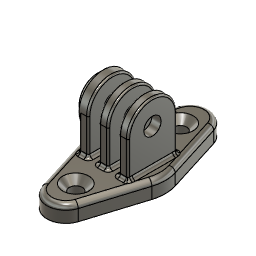
wall_mount (Autodesk Fusion 360 design; units mm, degrees)
Autodesk Fusion 360 part; units mm, degrees
sketch "Sketch3" plane through (0, 0, 0) normal (0, 1, 0) x (1, 0, 0)
  circle A0 centre (0, -16) radius 2
  circle A1 centre (0, 16) radius 2
  line L0 (-7, -16) -> (-12, 0)
  line L1 (-7, 16) -> (-12, 0)
  line L2 (7, -16) -> (12, 0)
  line L3 (7, 16) -> (12, 0)
  line L4 (-7, -16) -> (-5.5086, -20.7724)
  line L5 (7, -16) -> (5.5086, -20.7724)
  line L6 (-7, 16) -> (-5.5086, 20.7724)
  line L7 (7, 16) -> (5.5086, 20.7724)
  arc A2 (5.5086, 20.7724) -> (-5.5086, 20.7724) centre (0, 19.051) ccw
  arc A3 (-5.5086, -20.7724) -> (5.5086, -20.7724) centre (0, -19.051) ccw
  point P0 (0, -18)
  point P1 (0, -14)
  point P2 (0, 14)
  point P3 (0, 18)
  dimension "d1" = 5
  dimension "d2" = 5
  dimension "d3" = 5
  dimension "d4" = 5
  constraint coincident P1 A0
  constraint coincident P0 A0
  constraint coincident P3 A1
  constraint coincident P2 A1
  constraint parallel L0 L4
  constraint parallel L2 L5
  constraint parallel L1 L6
  constraint parallel L3 L7
  constraint tangent L6 A2
  constraint tangent L4 A3
  constraint tangent L5 A3
  measures "d1" distance of L0.start L4.end
  measures "d2" distance of L2.start L5.end
  measures "d3" distance of L1.start L6.end
  measures "d4" distance of L3.start L7.end
extrude "Extrude1" add sketch "Sketch3" along normal blind 5 makes body 1
fillet "Fillet1" radius 12 2 edges at (-12, 2.5, 0) (12, 2.5, 0) on bodies 1
sketch "Sketch5" plane through (1.4, 0, 0) normal (1, 0, 0) x (0, 0, -1)
  circle A0 centre (0, 16) radius 2.65
  line L0 (-3.5793, 5) -> (7.5, 5)
  line L1 (-3.5793, 5) -> (-7.5, 5)
  line L2 (-7.5, 16) -> (-7.5, 5)
  line L3 (7.5, 16) -> (7.5, 5)
  arc A1 (7.5, 16) -> (-7.5, 16) centre (0, 16) ccw
  point P0 (0, 18.65)
  point P1 (0, 13.35)
  point P2 (-3.5793, 5)
  constraint coincident P0 A0
  constraint coincident P1 A0
  constraint concentric A0 A1
  constraint coincident P2 L0.start
  constraint horizontal L0
  constraint parallel L0 L1
  constraint tangent L2 A1
  constraint perpendicular L1 L2
  constraint tangent L3 A1
extrude "Extrude2" add sketch "Sketch5" against normal blind 2.8 separate body makes body 2
copy_body "CopyPasteBodies1" bodies 2 makes body 3
move_body "Move3" bodies 3 to x (1, 0, 0) y (0, 1, 0) z (0, 0, 1) at (6.1, 0, 0)
copy_body "CopyPasteBodies2" bodies 2 makes body 4
move_body "Move4" bodies 4 to x (1, 0, 0) y (0, 1, 0) z (0, 0, 1) at (-6.1, 0, 0)
sketch "Sketch7" plane through (-7.5, 0, 0) normal (-1, 0, 0) x (0, 0, 1)
  line L0 (7.3, -0.8941) -> (1.5345, 8.6587)
  line L1 (1.5345, 8.6587) -> (0, -5.1088)
  line L2 (0, -5.1088) -> (7.3, -0.8941)
  circle A0 centre (0, 16) radius 7.5
  circle A1 centre (0, 16) radius 2.65
  point P0 (0, 16)
  dimension "d11" = 15
  constraint coincident P0 A0.centre
  measures "d11" diameter of A0
extrude "Extrude3" add sketch "Sketch7" along normal blind 2 separate body contours A0 makes body 5
sketch "Sketch8" plane through (-6.1, 0, 0) normal (-1, 0, 0) x (0, 0, 1)
  line L0 (-2.4537, 20.25) -> (-4.9075, 16)
  line L1 (-2.4537, 20.25) -> (-4.9075, 16)
  line L2 (-4.9075, 16) -> (-2.4537, 11.75)
  line L3 (-2.4537, 11.75) -> (2.4537, 11.75)
  line L4 (2.4537, 11.75) -> (4.9075, 16)
  line L5 (4.9075, 16) -> (2.4537, 20.25)
  line L6 (2.4537, 20.25) -> (-2.4537, 20.25)
  point P0 (-2.4537, 20.25)
  point P1 (2.4537, 20.25)
  point P2 (-4.9075, 16)
  point P3 (-2.4537, 11.75)
  point P4 (4.9075, 16)
  point P5 (2.4537, 11.75)
  constraint coincident P0 L0.start
  constraint coincident P2 L0.end
  constraint coincident P3 L2.end
  constraint coincident P5 L3.end
  constraint coincident P4 L4.end
  constraint coincident P1 L5.end
extrude "Extrude4" cut sketch "Sketch8" along normal blind 5 bodies 4 5
combine "Combine1" operation add target body 5 tool bodies 1 2 3 4
fillet "Fillet2" radius 1.5 8 edges at (-11.4277, 5, 0) (-8.195, 5, 12.1759) (0, 5, 24.8223) (8.195, 5, 12.1759) (11.4277, 5, 0) (8.195, 5, -12.1759) (0, 5, -24.8223) (-8.195, 5, -12.1759) on bodies 5
chamfer "Chamfer1" distance 2 angle 45 2 edges at (-1.8647, 5, -16.7232) (-1.8647, 5, 15.2768) on bodies 5
fillet "Fillet3" radius 0.5 17 edges at (7.5, 10.5, 7.5) (7.5, 23.5, 0) (7.5, 10.5, -7.5) (4.7, 10.5, 7.5) (4.7, 23.5, 0) (4.7, 10.5, -7.5) (1.4, 10.5, 7.5) (1.4, 23.5, 0) (1.4, 10.5, -7.5) (-1.4, 10.5, 7.5) (-1.4, 23.5, 0) (-1.4, 10.5, -7.5) (-4.7, 10.5, 7.5) (-4.7, 23.5, 0) (-4.7, 10.5, -7.5) (-7.5, 10.5, -7.5) (-7.5, 10.5, 7.5) on bodies 5
chamfer "Chamfer2" distance 2 angle 45 1 edges at (-9.5, 13.2879, -6.9925) on bodies 5
fillet "Fillet4" radius 0.5 1 edges at (-9.5, 17.9889, -5.1278) on bodies 5
fillet "Fillet5" radius 0.5 6 edges at (-9.5, 18.125, -3.6806) (-9.5, 20.25, 0) (-9.5, 18.125, 3.6806) (-9.5, 13.875, 3.6806) (-9.5, 11.75, 0) (-9.5, 13.875, -3.6806) on bodies 5
fillet "Fillet6" radius 1 24 edges at (-7.3536, 5, 7.3536) (-7.5, 5, 0) (-7.3536, 5, -7.3536) (-6.1, 5, -7.5) (-4.8464, 5, -7.3536) (-4.7, 5, 0) (-4.8464, 5, 7.3536) (-6.1, 5, 7.5) (-1.2536, 5, 7.3536) (-1.4, 5, 0) (-1.2536, 5, -7.3536) (0, 5, -7.5) (1.2536, 5, -7.3536) (1.4, 5, 0) (1.2536, 5, 7.3536) (0, 5, 7.5) (4.8464, 5, 7.3536) (4.7, 5, 0) (4.8464, 5, -7.3536) (6.1, 5, -7.5) (7.3536, 5, -7.3536) (7.5, 5, 0) (7.3536, 5, 7.3536) (6.1, 5, 7.5) on bodies 5
other "Base Mesh Feature2"
mesh_to_body "Convert Mesh2" makes body 6 makes body 7 makes body 8 makes body 9
sketch "Sketch2" plane through (0, 0, 0) normal (0, 1, 0) x (1, 0, 0)
other "Base Mesh Feature1"
mesh_to_body "Convert Mesh1" makes body 10 makes body 11 makes body 12 makes body 13
sketch "Sketch1" plane through (0, 0, 0) normal (0, 1, 0) x (1, 0, 0)
  line L0 (-0.0049, -0.0221) -> (0.0049, -0.0221)
  line L1 (0.0049, -0.0221) -> (0.0049, 0.0221)
  line L2 (0.0049, 0.0221) -> (-0.0049, 0.0221)
  line L3 (-0.0049, -0.0221) -> (-0.0049, 0.0221)
  point P0 (-0.0112, -0.0033)
  point P1 (-0.0049, -0.0221)
  point P2 (0.0049, -0.0221)
  point P3 (0.011, -0.0039)
  point P4 (-0.0112, 0.0033)
  point P5 (0.0113, 0.0025)
  point P6 (0.0049, 0.0221)
  point P7 (-0.0049, 0.0221)
  constraint coincident P1 L0.start
  constraint coincident P2 L0.end
  constraint coincident P6 L1.end
  constraint coincident P7 L2.end
named bodies: "bracket", "bracket (1)", "bracket (2)", "bracket (3)"
